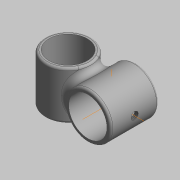
# Autodesk Inventor part: L45-6
Saved by Autodesk Inventor 2019.4 (Build 234330000, 330)
## iProperties
Created: 2020-04-23
Part Number: L45-6
Material: Generic
Document SubType Name: Modeling
Designer: Hannah
Density: 1 g/cm^3
Appearance: Default
Author: Hannah
Autodesk Inventor part; units mm, degrees
ref_plane "XZ Plane" through (0, 0, 0) normal (0, 1, 0) x (-1, 0, 0)
ref_plane "XY Plane" through (0, 0, 0) normal (0, 0, 1) x (1, 0, 0)
sketch "Sketch1" plane through (0, 0, 0) normal (0, 0, 1) x (1, 0, 0)
  circle A0 centre (0, 0) radius 17.5
  circle A1 centre (0, 0) radius 21
  dimension "d1" = 42
  dimension "d2" = 35
  constraints: 2 centre point, 2 coincident
  measures "d1" diameter of A1
  measures "d2" diameter of A0
extrude "Extrusion1" add sketch "Sketch1" along normal mid plane 44 contours A0 | A1
sketch "Sketch2" plane through (0, 0, 0) normal (0, 1, 0) x (-1, 0, 0)
  circle A0 centre (40, 0) radius 17.5
  circle A1 centre (40, 0) radius 21
  line L0 (77.9619, 0) -> (-37.4937, 0) projected
  line L1 (0, -30.8) -> (0, 30.8) projected
  point P0 (0, 0)
  dimension "d5" = 35
  dimension "d6" = 42
  dimension "d13" = 40
  constraints: 2 centre point, 1 coincident, 1 point on line
  measures "d5" diameter of A0
  measures "d6" diameter of A1
  measures "d13" distance from line of L1 A0.centre
extrude "Extrusion2" add sketch "Sketch2" along normal mid plane 44
fillet "Fillet1" radius 5 4 edges at (-20, 6.4031, 6.4031) (-20, 6.4031, -6.4031) (-20, -6.4031, -6.4031) (-20.0001, -6.403, 6.4033)
extrude "Extrusion3" cut sketch "Sketch2" along normal through all both and the other way through all contours L0 A0 | A0 L0
extrude "Extrusion4" cut sketch "Sketch1" along normal through all both and the other way through all contours A0
hole "Hole1" at (0, 0, 0) direction (1, 0, 0) diameter 6.647 end through all thread size "M8x1.25" class "6H" standard "ISO Metric profile"
ref_plane "Work Plane1" through (-40, 0, 0) normal (1, 0, 0) x (0, 1, 0)
hole "Hole2" at (-40, 0, 0) direction (-1, 0, 0) diameter 6.647 end through all thread size "M8x1.25" class "6H" standard "ISO Metric profile"
fillet "Fillet2" radius 2 4 edges at (-19, 22, 0) (-19, -22, 0) (-21, 0, 22) (-21, 0, -22)
equation "\"d5\" = d2"
equation "\"d6\" = d1"
equation "\"d7\" = d3"
equation "\"d3\" = 44"
body "Solid1"
